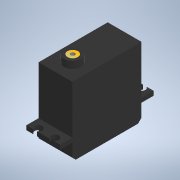
# Autodesk Inventor part: Motor
Saved by Autodesk Inventor 2020 (Build 240168000, 168)
## iProperties
Created: 2019-09-17
Part Number: Motor
Material: 일반
Document SubType Name: Modeling
Designer: Knowblesse
Density: 1 g/cm^3
Appearance: 기본값
Author: Knowblesse
Autodesk Inventor part; units mm, degrees
ref_plane "YZ Plane" through (0, 0, 0) normal (1, 0, 0) x (0, 1, 0)
ref_plane "XZ Plane" through (0, 0, 0) normal (0, 1, 0) x (-1, 0, 0)
ref_plane "XY Plane" through (0, 0, 0) normal (0, 0, 1) x (1, 0, 0)
sketch "스케치1" plane through (0, 0, 0) normal (0, 0, 1) x (1, 0, 0)
  line L0 (0, 0) -> (19.5, 0)
  line L1 (19.5, 0) -> (19.5, 40)
  line L2 (19.5, 40) -> (0, 40)
  line L3 (0, 40) -> (0, 0)
  dimension "d0" = 19.5
  dimension "d1" = 40
  constraints: 8 end point, 2 parallel, 1 horizontal, 1 perpendicular
  measures "d0" distance of L2.end L1.end
  measures "d1" distance of L1.end L0.end
extrude "돌출1" add sketch "스케치1" along normal blind 40
sketch "스케치2" plane through (0, 40, 0) normal (0, 1, 0) x (1, 0, 0)
  line L0 (19.5, 0) -> (0, 0) projected
  line L1 (0, 0) -> (0, -40) projected
  line L2 (19.5, -40) -> (0, -40) projected
  line L3 (19.5, 0) -> (19.5, -40) projected
  circle A0 centre (9.75, -30) radius 5
  point P0 (9.75, -40)
  dimension "d4" = 10
  dimension "d5" = 10
  constraints: 1 centre point, 1 coincident, 1 midpoint, 1 vertical alignment
  measures "d4" distance from line of L2 point (9.75, -30)
  measures "d5" diameter of A0
extrude "돌출2" add sketch "스케치2" along normal blind 4 contours A0
sketch "스케치3" plane through (9.75, 44, 30) normal (0, 1, 0) x (1, 0, 0)
  circle A0 centre (0, 0) radius 3
  point P0 (-9.75, 30)
  dimension "d8" = 6
  constraints: 1 centre point
  measures "d8" diameter of A0
extrude "돌출3" cut sketch "스케치3" against normal blind 4
sketch "스케치4" plane through (9.75, 40, 30) normal (0, 1, 0) x (1, 0, 0)
  circle A0 centre (0, 0) radius 3 projected
  point P0 (-9.75, 30)
extrude "돌출4" add sketch "스케치4" along normal blind 4 separate body
sketch "스케치5" plane through (9.75, 44, 30) normal (0, 1, 0) x (1, 0, 0)
  circle A0 centre (0, 0) radius 3 projected
  point P0 (-9.75, 30)
hole "구멍1" at (9.75, 44, 30) direction (0, -1, 0) diameter 2.459 depth 4 bodies 2 thread size "M3x0.5" class "6H" standard "ANSI Metric M Profile"
sketch "스케치6" plane through (0, 0, 0) normal (0, -1, 0) x (1, 0, 0)
  circle A0 centre (9.75, 30) radius 1.2295 projected
  circle A1 centre (9.75, 30) radius 5 projected
  circle A2 centre (9.75, 30) radius 7
  point P0 (0, 0)
  dimension "d20" = 14
  constraints: 1 centre point, 1 coincident
  measures "d20" diameter of A2
extrude "돌출5" add sketch "스케치6" along normal blind 2 contours A1 | A2 bodies 1
chamfer "모따기1" distance 2 angle 45 1 edges at (2.75, -2, 30)
chamfer "모따기2" distance 2 angle 45 2 edges at (9.75, 0, 40) (9.75, 0, 0)
sketch "스케치9" plane through (0, 0, 40) normal (0, 0, 1) x (1, 0, 0)
  line L0 (19.5, 2) -> (19.5, 40) projected
  line L1 (0, 40) -> (0, 2) projected
  line L2 (19.5, 12) -> (0, 12)
  line L3 (0, 12) -> (0, 9.5)
  line L4 (0, 9.5) -> (19.5, 9.5)
  line L5 (19.5, 9.5) -> (19.5, 12)
  line L6 (19.5, 40) -> (0, 40) projected
  point P0 (0, 0)
  point P1 (0, 12)
  dimension "d34" = 2.5
  dimension "d35" = 28
  constraints: 8 end point, 2 parallel, 2 point on line, 1 horizontal, 1 perpendicular
  measures "d34" distance of L3.end L2.end
  measures "d35" distance between parallel lines of L2 L6
extrude "돌출8" add sketch "스케치9" along normal blind 7 contours L4 L1 L2 L0 bodies 1
sketch "스케치10" plane through (0, 0, 0) normal (0, 0, -1) x (-1, 0, 0)
  line L0 (0, 12) -> (0, 9.5) projected
  line L1 (0, 9.5) -> (-19.5, 9.5) projected
  line L2 (-19.5, 9.5) -> (-19.5, 12) projected
  line L3 (-19.5, 12) -> (0, 12) projected
  point P0 (0, 0)
extrude "돌출9" add sketch "스케치10" along normal blind 7 bodies 1
sketch "스케치12" plane through (0, 9.5, 40) normal (0, -1, 0) x (1, 0, 0)
  line L0 (19.5, 0) -> (0, 0) projected
  line L1 (19.5, 0) -> (19.5, 7) projected
  line L2 (0, 7) -> (19.5, 7) projected
  line L3 (0, 0) -> (0, 7) projected
  line L4 (0, -40) -> (19.5, -40) projected
  line L5 (0, -40) -> (0, -47) projected
  line L6 (19.5, -47) -> (0, -47) projected
  line L7 (19.5, -40) -> (19.5, -47) projected
  point P0 (0, -40)
  point P1 (14.5, 5)
  point P2 (5, 5)
  point P3 (14.5, -45)
  point P4 (5, -45)
  dimension "d40" = 2
  dimension "d41" = 2
  dimension "d42" = 5
  dimension "d43" = 5
  constraints: 2 horizontal alignment, 2 vertical alignment
  measures "d40" distance from line of L2 point (14.5, 5)
  measures "d41" distance from line of point (14.5, -45) L6
  measures "d42" distance from line of L1 point (14.5, 5)
  measures "d43" distance from line of point (5, 5) L3
hole "구멍2" at (14.5, 9.5, 45) at (5, 9.5, 45) at (5, 9.5, -5) at (14.5, 9.5, -5) direction (0, 1, 0) diameter 4.5 end through all bodies 1
